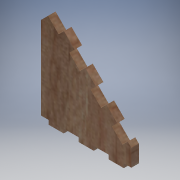
# Autodesk Inventor part: SledSideSupport
Saved by Autodesk Inventor 2019 (Build 230136000, 136)
## iProperties
Created: 2019-01-14
Part Number: SledSideSupport
Material: Wood (Birch)
Document SubType Name: Modeling
Designer: nxgam
Density: 0.55 g/cm^3
Appearance: Birch - Natural Polished
Author: nxgam
Autodesk Inventor part; units mm, degrees
ref_plane "YZ Plane" through (0, 0, 0) normal (1, 0, 0) x (0, 1, 0)
ref_plane "XZ Plane" through (0, 0, 0) normal (0, 1, 0) x (-1, 0, 0)
ref_plane "XY Plane" through (0, 0, 0) normal (0, 0, 1) x (1, 0, 0)
sketch "Sketch1" plane through (0, 0, 0) normal (0, 0, 1) x (1, 0, 0)
  line L0 (0, 0) -> (60.96, 0)
  line L1 (60.96, 0) -> (60.96, 2.794) construction
  line L2 (60.96, 101.6) -> (0, 101.6)
  line L3 (0, 101.6) -> (0, 2.794)
  line L4 (-5.08, 0) -> (5.08, 0)
  line L5 (5.08, 0) -> (5.08, 2.794)
  line L6 (5.08, 2.794) -> (-5.08, 2.794)
  line L7 (-5.08, 2.794) -> (-5.08, 0) construction
  line L8 (15.24, 0) -> (25.4, 0)
  line L9 (25.4, 0) -> (25.4, 2.794)
  line L10 (25.4, 2.794) -> (15.24, 2.794)
  line L11 (15.24, 2.794) -> (15.24, 0)
  line L12 (35.56, 0) -> (45.72, 0)
  line L13 (45.72, 0) -> (45.72, 2.794)
  line L14 (45.72, 2.794) -> (35.56, 2.794)
  line L15 (35.56, 2.794) -> (35.56, 0)
  line L16 (55.88, 0) -> (66.04, 0) construction
  line L17 (66.04, 0) -> (66.04, 2.794) construction
  line L18 (66.04, 2.794) -> (55.88, 2.794)
  line L19 (55.88, 2.794) -> (55.88, 0)
  line L20 (60.96, 2.794) -> (60.96, 101.6)
  line L21 (0, 2.794) -> (0, 0) construction
  line L22 (0, 2.794) -> (5.08, 2.794)
  line L23 (5.08, 0) -> (5.08, 2.794)
  line L24 (5.08, 0) -> (15.24, 0)
  line L25 (15.24, 0) -> (15.24, 2.794)
  line L26 (15.24, 2.794) -> (25.4, 2.794)
  line L27 (25.4, 2.794) -> (25.4, 0)
  line L28 (25.4, 0) -> (35.56, 0)
  line L29 (35.56, 0) -> (35.56, 2.794)
  line L30 (35.56, 2.794) -> (45.72, 2.794)
  line L31 (45.72, 2.794) -> (45.72, 0)
  line L32 (45.72, 0) -> (55.88, 0)
  line L33 (55.88, 0) -> (55.88, 2.794)
  line L34 (55.88, 2.794) -> (60.96, 2.794)
  dimension "d0" = 10.16
  dimension "d1" = 2.794
  dimension "d5" = 20.32
  dimension "d11" = 101.6
  dimension "d14" = 5.08
  dimension "d15" = 5.08
  constraints: 70 end point, 11 perpendicular, 7 parallel, 4 collinear, 4 horizontal, 2 midpoint, 1 point on line, 24 other
  measures "d0" distance of L5.end L6.end
  measures "d1" distance of L4.end L5.end
  measures "d5" distance of L4.start L8.start
  measures "d11" distance between parallel lines of L0 L2
  measures "d14" distance between parallel lines of L7 L3
  measures "d15" distance between parallel lines of L1 L19
extrude "Extrusion2" add sketch "Sketch1" along normal blind 5.08 contours L5 L6 L3 L2 L20 L18 L19 L0 L13 L14 L15 L9 L10 L11
sketch "Sketch2" plane through (0, 0, 5.08) normal (0, 0, 1) x (1, 0, 0)
  line L0 (33.3926, 34.8025) -> (40.5768, 27.6183) projected
  line L1 (36.9847, 38.3946) -> (44.1689, 31.2104) projected
  line L2 (58.5374, 16.8419) -> (61.3536, 14.0257)
  line L3 (61.3536, 14.0257) -> (94.79, 106.8091)
  line L4 (94.79, 106.8091) -> (9.0512, 130.8761)
  line L5 (9.0512, 130.8761) -> (-6.9479, 112.9626)
  line L6 (-6.9479, 112.9626) -> (0, 75.3793)
  line L7 (0, 101.6) -> (0, 2.794) projected
  line L8 (0, 75.3793) -> (58.5374, 16.8419)
  line L9 (36.9847, 38.3946) -> (33.3926, 34.8025) projected
  line L10 (40.5768, 27.6183) -> (44.1689, 31.2104) projected
  point P0 (0, 0)
  constraints: 12 end point, 3 point on line
extrude "Extrusion3" cut sketch "Sketch2" against normal blind 5.08 contours L8 L6 L5 L4 L3 L2 L1
sketch "Sketch3" plane through (0, 0, 5.08) normal (0, 0, 1) x (1, 0, 0)
  line L0 (33.3926, 34.8025) -> (40.5768, 27.6183) projected
  line L1 (36.9847, 38.3946) -> (44.1689, 31.2104) projected
  line L2 (60.96, 14.4193) -> (0, 75.3793) projected
  line L3 (58.5374, 16.8419) -> (51.3531, 24.0262)
  line L4 (51.3531, 24.0262) -> (47.761, 20.434)
  line L5 (47.761, 20.434) -> (54.9452, 13.2498)
  line L6 (54.9452, 13.2498) -> (58.5374, 16.8419)
  line L7 (44.1689, 31.2104) -> (36.9847, 38.3946)
  line L8 (36.9847, 38.3946) -> (33.3926, 34.8025)
  line L9 (33.3926, 34.8025) -> (40.5768, 27.6183)
  line L10 (40.5768, 27.6183) -> (44.1689, 31.2104)
  line L11 (29.8005, 45.5788) -> (22.6163, 52.763)
  line L12 (22.6163, 52.763) -> (19.0242, 49.1709)
  line L13 (19.0242, 49.1709) -> (26.2084, 41.9867)
  line L14 (26.2084, 41.9867) -> (29.8005, 45.5788)
  line L15 (15.4321, 59.9472) -> (8.2479, 67.1314)
  line L16 (8.2479, 67.1314) -> (4.6558, 63.5393)
  line L17 (4.6558, 63.5393) -> (11.84, 56.3551)
  line L18 (11.84, 56.3551) -> (15.4321, 59.9472)
  line L19 (1.0637, 74.3156) -> (-6.1205, 81.4998)
  line L20 (-6.1205, 81.4998) -> (-9.7126, 77.9077)
  line L21 (-9.7126, 77.9077) -> (-2.5284, 70.7235)
  line L22 (-2.5284, 70.7235) -> (1.0637, 74.3156)
  line L23 (-13.3047, 88.684) -> (-20.4889, 95.8682)
  line L24 (-20.4889, 95.8682) -> (-24.081, 92.2761)
  line L25 (-24.081, 92.2761) -> (-16.8968, 85.0919)
  line L26 (-16.8968, 85.0919) -> (-13.3047, 88.684)
  line L27 (36.9847, 38.3946) -> (33.3926, 34.8025) projected
  line L28 (40.5768, 27.6183) -> (44.1689, 31.2104) projected
  point P0 (0, 0)
  point P1 (46.5916, 28.7877)
  point P2 (26.2084, 41.9867)
  point P3 (32.2232, 43.1561)
  point P4 (11.84, 56.3551)
  point P5 (17.8548, 57.5245)
  point P6 (-2.5284, 70.7235)
  point P7 (3.4864, 71.8929)
  point P8 (-16.8968, 85.0919)
  point P9 (-10.882, 86.2613)
  dimension "d24" = 20.32
  dimension "d20" = 5.08
  constraints: 48 end point, 2 parallel, 1 perpendicular, 1 point on line, 50 other
  measures "d20" distance of L3.end L4.end
extrude "Extrusion4" cut sketch "Sketch3" against normal blind 5.08 contours L8 L1 L10 L0 | L22 L21 L20 L19 L2 | L18 L17 L16 L2 | L14 L13 L12 L2 | L2 L6 L5 L4
sketch "Sketch4" plane through (0, 0, 5.08) normal (0, 0, 1) x (1, 0, 0)
  line L0 (4.6558, 63.5393) -> (8.2479, 67.1314) projected
  line L1 (8.2479, 67.1314) -> (1.0637, 74.3156) projected
  line L2 (1.0637, 74.3156) -> (0, 73.2519) projected
  line L3 (0, 73.2519) -> (0, 2.794) construction
  line L4 (0, 2.794) -> (5.08, 2.794) projected
  line L5 (5.08, 2.794) -> (5.08, 0) projected
  line L6 (5.08, 0) -> (15.24, 0) projected
  line L7 (15.24, 0) -> (15.24, 2.794) projected
  line L8 (15.24, 2.794) -> (25.4, 2.794) projected
  line L9 (25.4, 2.794) -> (25.4, 0) projected
  line L10 (25.4, 0) -> (35.56, 0) projected
  line L11 (35.56, 0) -> (35.56, 2.794) projected
  line L12 (35.56, 2.794) -> (45.72, 2.794) projected
  line L13 (45.72, 2.794) -> (45.72, 0) projected
  line L14 (45.72, 0) -> (55.88, 0) projected
  line L15 (55.88, 0) -> (55.88, 2.794) projected
  line L16 (55.88, 2.794) -> (60.96, 2.794) projected
  line L17 (60.96, 2.794) -> (60.96, 14.4193) projected
  line L18 (60.96, 14.4193) -> (58.5374, 16.8419) projected
  line L19 (58.5374, 16.8419) -> (54.9452, 13.2498) projected
  line L20 (54.9452, 13.2498) -> (47.761, 20.434) projected
  line L21 (47.761, 20.434) -> (51.3531, 24.0262) projected
  line L22 (51.3531, 24.0262) -> (44.1689, 31.2104) projected
  line L23 (44.1689, 31.2104) -> (40.5768, 27.6183) projected
  line L24 (40.5768, 27.6183) -> (33.3926, 34.8025) projected
  line L25 (33.3926, 34.8025) -> (36.9847, 38.3946) projected
  line L26 (36.9847, 38.3946) -> (29.8005, 45.5788) projected
  line L27 (29.8005, 45.5788) -> (26.2084, 41.9867) projected
  line L28 (26.2084, 41.9867) -> (19.0242, 49.1709) projected
  line L29 (19.0242, 49.1709) -> (22.6163, 52.763) projected
  line L30 (22.6163, 52.763) -> (15.4321, 59.9472) projected
  line L31 (15.4321, 59.9472) -> (11.84, 56.3551) projected
  line L32 (11.84, 56.3551) -> (4.6558, 63.5393) projected
  line L33 (4.6558, 63.5393) -> (0, 58.8835)
  line L34 (0, 73.2519) -> (0, 2.794) construction
  line L35 (4.6558, 63.5393) -> (8.2479, 67.1314)
  line L36 (8.2479, 67.1314) -> (3.9736, 83.8978)
  line L37 (3.9736, 83.8978) -> (-8.4485, 80.2357)
  line L38 (-8.4485, 80.2357) -> (0, 58.8835)
  line L39 (4.6558, 63.5393) -> (8.2479, 67.1314) projected
  line L40 (8.2479, 67.1314) -> (3.9736, 83.8978)
  line L41 (0, 58.8835) -> (8.2479, 67.1314)
  line L42 (0, 58.8835) -> (-8.4485, 80.2357)
  point P0 (0, 0)
  constraints: 16 end point, 3 collinear, 1 point on line
extrude "Extrusion5" cut sketch "Sketch4" against normal blind 5.08
equation "\"d5\" = 2 * d0"
equation "\"d24\" = 2 * d21"
equation "\"d21\" = 10.16"
body "Solid2"
